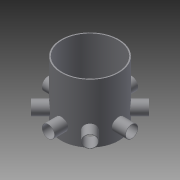
# Autodesk Inventor part: Vacuum Cylinder
Saved by Autodesk Inventor 2015 (Build 190159000, 159)
## iProperties
Created: 2014-05-19
Part Number: Vacuum Cylinder
Material: Generic
Document SubType Name: Modeling
Designer: ijs09
Density: 1 g/cm^3
Appearance: Default
Author: ijs09
Autodesk Inventor part; units mm, degrees
note: some values were not read from the file. Chosen so that the rebuilt part matches the saved one: second side of "Extrusion1".
sketch "Sketch1" plane through (0, 0, 0) normal (0, 0, 1) x (1, 0, 0)
  circle A0 centre (0, 0) radius 97.6
  circle A1 centre (0, 0) radius 101.6
  dimension "d0" = 195.2
  dimension "d1" = 203.2
  constraints: 2 centre point, 2 coincident
  measures "d0" diameter of A0
  measures "d1" diameter of A1
extrude "Extrusion1" add sketch "Sketch1" along normal blind 206.6
ref_plane "Work Plane1" through (0, -101.6, 0) normal (0, 1, 0) x (-1, 0, 0)
ref_plane "Work Plane2" through (0, 101.6, 0) normal (0, 1, 0) x (-1, 0, 0)
ref_plane "Work Plane3" through (-101.6, 0, 0) normal (1, 0, 0) x (0, 1, 0)
ref_plane "Work Plane4" through (101.6, 0, 0) normal (1, 0, 0) x (0, 1, 0)
sketch "Sketch2" plane through (0, -101.6, 0) normal (0, 1, 0) x (-1, 0, 0)
  circle A0 centre (0, 50.3) radius 22.35
  line L0 (-101.6, 0) -> (101.6, 0) projected
  point P0 (0, 0)
  dimension "d4" = 44.7
  dimension "d5" = 50.3
  constraints: 1 centre point
  measures "d4" diameter of A0
  measures "d5" distance from line of A0.centre L0
extrude "Extrusion2" add sketch "Sketch2" against normal blind 45
sketch "Sketch3" plane through (0, -101.6, 0) normal (0, 1, 0) x (-1, 0, 0)
  circle A0 centre (0, 50.3) radius 22.35
  line L0 (-101.6, 0) -> (101.6, 0) projected
  point P0 (0, 0)
  dimension "d8" = 44.7
  dimension "d116" = 50.3
  constraints: 1 centre point
  measures "d8" diameter of A0
  measures "d116" distance from line of A0.centre L0
extrude "Extrusion3" add sketch "Sketch3" along normal up to next
sketch "Sketch4" plane through (101.6, 0, 0) normal (1, 0, 0) x (0, 1, 0)
  circle A0 centre (0, 50.3) radius 22.35
  line L0 (-101.6, 0) -> (101.6, 0) projected
  point P0 (0, 0)
  dimension "d12" = 44.7
  dimension "d13" = 50.3
  constraints: 1 centre point
  measures "d12" diameter of A0
  measures "d13" distance from line of A0.centre L0
extrude "Extrusion4" add sketch "Sketch4" along normal blind 45
sketch "Sketch5" plane through (101.6, 0, 0) normal (1, 0, 0) x (0, 1, 0)
  circle A0 centre (0, 50.3) radius 22.35
  line L0 (-101.6, 0) -> (101.6, 0) projected
  point P0 (0, 0)
  dimension "d16" = 44.7
  dimension "d117" = 50.3
  constraints: 1 centre point
  measures "d16" diameter of A0
  measures "d117" distance from line of A0.centre L0
extrude "Extrusion5" add sketch "Sketch5" against normal up to next
sketch "Sketch6" plane through (0, 101.6, 0) normal (0, 1, 0) x (-1, 0, 0)
  circle A0 centre (0, 50.3) radius 22.35
  line L0 (-101.6, 0) -> (101.6, 0) projected
  point P0 (0, 0)
  dimension "d22" = 44.7
  dimension "d23" = 50.3
  constraints: 1 centre point
  measures "d22" diameter of A0
  measures "d23" distance from line of A0.centre L0
extrude "Extrusion6" add sketch "Sketch6" along normal blind 45
sketch "Sketch7" plane through (0, 101.6, 0) normal (0, 1, 0) x (-1, 0, 0)
  circle A0 centre (0, 50.3) radius 22.35
  line L0 (-101.6, 0) -> (101.6, 0) projected
  point P0 (0, 0)
  dimension "d26" = 44.7
  dimension "d118" = 50.3
  constraints: 1 centre point
  measures "d26" diameter of A0
  measures "d118" distance from line of A0.centre L0
extrude "Extrusion7" add sketch "Sketch7" against normal up to next
sketch "Sketch8" plane through (-101.6, 0, 0) normal (1, 0, 0) x (0, 1, 0)
  circle A0 centre (0, 50.3) radius 22.35
  line L0 (-101.6, 0) -> (101.6, 0) projected
  point P0 (0, 0)
  dimension "d32" = 44.7
  dimension "d33" = 50.3
  constraints: 1 centre point
  measures "d32" diameter of A0
  measures "d33" distance from line of A0.centre L0
extrude "Extrusion8" add sketch "Sketch8" against normal blind 45
sketch "Sketch9" plane through (-101.6, 0, 0) normal (1, 0, 0) x (0, 1, 0)
  circle A0 centre (0, 50.3) radius 22.35
  line L0 (-101.6, 0) -> (101.6, 0) projected
  point P0 (0, 0)
  dimension "d36" = 44.7
  dimension "d119" = 50.3
  constraints: 1 centre point
  measures "d36" diameter of A0
  measures "d119" distance from line of A0.centre L0
extrude "Extrusion9" add sketch "Sketch9" along normal up to next
hole "Hole1" at (-146.6, 0, 50.3) direction (1, 0, 0) diameter 41.4 depth 100
hole "Hole2" at (146.6, 0, 50.3) direction (-1, 0, 0) diameter 41.8 depth 100
hole "Hole3" at (0, -146.6, 50.3) direction (0, 1, 0) diameter 42.5 end through all
ref_plane "Work Plane5" through (0, 0, 0) normal (-0.7071068, 0.7071068, 0) x (0, 0, 1)
ref_plane "Work Plane6" through (-71.842, 71.842, 0) normal (-0.7071068, 0.7071068, 0) x (-0.7071068, -0.7071068, 0)
sketch "Sketch10" plane through (-71.842, 71.842, 0) normal (-0.7071068, 0.7071068, 0) x (-0.7071068, -0.7071068, 0)
  circle A0 centre (0, 50.3) radius 22.35
  line L0 (-101.6, 0) -> (101.6, 0) projected
  point P0 (0, 0)
  dimension "d69" = 44.7
  dimension "d70" = 50.3
  constraints: 1 centre point
  measures "d69" diameter of A0
  measures "d70" distance from line of A0.centre L0
extrude "Extrusion10" add sketch "Sketch10" along normal blind 45
sketch "Sketch11" plane through (-71.842, 71.842, 0) normal (-0.7071068, 0.7071068, 0) x (-0.7071068, -0.7071068, 0)
  circle A0 centre (0, 50.3) radius 22.35
  line L0 (-101.6, 0) -> (101.6, 0) projected
  point P0 (0, 0)
  dimension "d73" = 44.7
  dimension "d120" = 50.3
  constraints: 1 centre point
  measures "d73" diameter of A0
  measures "d120" distance from line of A0.centre L0
extrude "Extrusion11" add sketch "Sketch11" against normal up to next
hole "Hole4" at (-103.6619, 103.6619, 50.3) direction (0.7071068, -0.7071068, 0) diameter 41.4 depth 100
ref_plane "Work Plane7" through (0, 0, 0) normal (0.7071068, 0.7071068, 0) x (0, 0, 1)
ref_plane "Work Plane8" through (-71.842, -71.842, 0) normal (0.7071068, 0.7071068, 0) x (-0.7071068, 0.7071068, 0)
sketch "Sketch12" plane through (-71.842, -71.842, 0) normal (0.7071068, 0.7071068, 0) x (-0.7071068, 0.7071068, 0)
  circle A0 centre (0, 50.3) radius 22.35
  line L0 (-101.6, 0) -> (101.6, 0) projected
  point P0 (0, 0)
  dimension "d89" = 44.7
  dimension "d90" = 50.3
  constraints: 1 centre point
  measures "d89" diameter of A0
  measures "d90" distance from line of A0.centre L0
extrude "Extrusion12" add sketch "Sketch12" against normal blind 45
sketch "Sketch13" plane through (-71.842, -71.842, 0) normal (0.7071068, 0.7071068, 0) x (-0.7071068, 0.7071068, 0)
  circle A0 centre (0, 50.3) radius 22.35
  line L0 (-101.6, 0) -> (101.6, 0) projected
  point P0 (0, 0)
  dimension "d93" = 44.7
  dimension "d121" = 50.3
  constraints: 1 centre point
  measures "d93" diameter of A0
  measures "d121" distance from line of A0.centre L0
extrude "Extrusion13" add sketch "Sketch13" along normal up to next
hole "Hole5" at (-103.6619, -103.6619, 50.3) direction (0.7071068, 0.7071068, 0) diameter 41.4 depth 100
sketch "Sketch14" plane through (0, 0, 0) normal (0, 0, -1) x (-1, 0, 0)
  point P0 (0, 0)
ref_plane "Work Plane9" through (0, 0, 20) normal (0, 0, 1) x (1, 0, 0)
ref_plane "Work Plane10" through (71.842, -71.842, 0) normal (-0.7071068, 0.7071068, 0) x (0, 0, 1)
sketch "Sketch16" plane through (71.842, -71.842, 0) normal (-0.7071068, 0.7071068, 0) x (0, 0, 1)
  circle A0 centre (50.3, 0) radius 22.35 projected
  circle A1 centre (50.3, 0) radius 22.35
  point P0 (0, 0)
  dimension "d134" = 44.7
  constraints: 1 centre point, 1 coincident
  measures "d134" diameter of A1
extrude "Extrusion16" add sketch "Sketch16" along normal up to next
sketch "Sketch17" plane through (71.842, -71.842, 0) normal (0.7071068, -0.7071068, 0) x (-0.7071068, -0.7071068, 0)
  circle A0 centre (0, -50.3) radius 22.35
  line L0 (101.6, 10) -> (-101.6, 10) projected
  point P0 (0, 0)
  dimension "d137" = 44.7
  dimension "d174" = 50.3
  constraints: 1 centre point
  measures "d137" diameter of A0
  measures "d174" distance of point (0, 0) A0.centre
extrude "Extrusion17" add sketch "Sketch17" along normal blind 45
sketch "Sketch18" plane through (103.6619, -103.6619, 50.3) normal (0.7071068, -0.7071068, 0) x (-0.7071068, -0.7071068, 0)
  circle A0 centre (0, 0) radius 21.25
  point P0 (0, 50.3)
  dimension "d141" = 42.5
  constraints: 1 centre point
  measures "d141" diameter of A0
hole "Hole6" at (103.6619, -103.6619, 50.3) direction (-0.7071068, 0.7071068, 0) diameter 41.4 depth 50 tip angle 118
ref_plane "Work Plane11" through (71.842, 71.842, 0) normal (0.7071068, 0.7071068, 0) x (0, 0, 1)
sketch "Sketch19" plane through (71.842, 71.842, 0) normal (0.7071068, 0.7071068, 0) x (0, 0, 1)
  circle A0 centre (50.3, 0) radius 22.35
  line L0 (-10, 101.6) -> (-10, -101.6) projected
  point P0 (0, 0)
  dimension "d150" = 44.7
  dimension "d175" = 50.3
  constraints: 1 centre point
  measures "d150" diameter of A0
  measures "d175" distance of point (0, 0) A0.centre
extrude "Extrusion18" add sketch "Sketch19" against normal up to next
sketch "Sketch20" plane through (71.842, 71.842, 0) normal (0.7071068, 0.7071068, 0) x (-0.7071068, 0.7071068, 0)
  circle A0 centre (0, 50.3) radius 22.35
  line L0 (-101.6, -10) -> (101.6, -10) projected
  line L1 (-101.6, 0) -> (101.6, 0) projected
  point P0 (0, 0)
  dimension "d154" = 44.7
  dimension "d176" = 50.3
  constraints: 1 centre point
  measures "d154" diameter of A0
  measures "d176" distance from line of L1 A0.centre
extrude "Extrusion19" add sketch "Sketch20" along normal blind 45
sketch "Sketch21" plane through (103.6619, 103.6619, 50.3) normal (0.7071068, 0.7071068, 0) x (-0.7071068, 0.7071068, 0)
  circle A0 centre (0, 0) radius 21.25
  point P0 (0, -50.3)
  dimension "d158" = 42.5
  constraints: 1 centre point
  measures "d158" diameter of A0
hole "Hole7" at (103.6619, 103.6619, 50.3) direction (-0.7071068, -0.7071068, 0) diameter 41.4 depth 52
equation "\"d8\" = d4"
equation "\"d116\" = d5"
equation "\"d12\" = d4"
equation "\"d13\" = d5"
equation "\"d16\" = d4"
equation "\"d117\" = d5"
equation "\"d22\" = d4"
equation "\"d23\" = d5"
equation "\"d26\" = d4"
equation "\"d118\" = d5"
equation "\"d33\" = d5"
equation "\"d119\" = d5"
equation "\"d69\" = d4"
equation "\"d70\" = d5"
equation "\"d73\" = d4"
equation "\"d120\" = d5"
equation "\"d89\" = d4"
equation "\"d90\" = d5"
equation "\"d93\" = d4"
equation "\"d121\" = d5"
body "Solid1"
